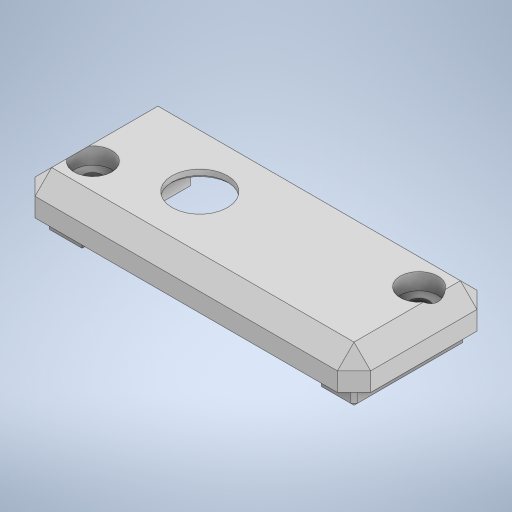
# Autodesk Inventor part: Arm_3_b
Saved by Autodesk Inventor 2023 (Build 270158000, 158)
## iProperties
Created: 2025-02-13
Part Number: Arm_3_b
Material: Generic
Document SubType Name: Modeling
Designer: Swoby
Density: 1 g/cm^3
Appearance: Default
Author: Swoby
Autodesk Inventor part; units mm, degrees
sketch "Sketch1" plane through (0, 0, 0) normal (0, 0, 1) x (1, 0, 0)
  line L0 (0, 0) -> (0, 3.1)
  line L1 (0, 3.1) -> (-5, 3.1)
  line L2 (-5, 3.1) -> (-5, 1.5)
  line L3 (-5, 1.5) -> (-7.4, 1.5)
  line L4 (-7.4, 1.5) -> (-7.4, 0)
  line L5 (-7.4, 0) -> (0, 0)
  line L6 (-7.4, 0) -> (-10.65, 0)
  line L7 (-10.65, 0) -> (-10.65, -7.1)
  line L8 (-10.65, -7.1) -> (-18.15, -7.1)
  line L9 (-18.15, -7.1) -> (-18.15, -10.8)
  line L10 (-18.15, -10.8) -> (-10.65, -10.8)
  line L11 (-10.65, -10.8) -> (-10.65, -31.3)
  line L12 (-10.65, -31.3) -> (-20.15, -31.3)
  line L13 (-20.15, -31.3) -> (-20.15, -36.7)
  line L14 (-20.15, -36.7) -> (-10.65, -36.7)
  line L15 (-10.65, -36.7) -> (-10.65, -40.6)
  line L16 (-10.65, -40.6) -> (30.95, -40.6)
  line L17 (30.95, -40.6) -> (30.95, -10.8)
  line L18 (30.95, -10.8) -> (38.45, -10.8)
  line L19 (38.45, -10.8) -> (38.45, -7.1)
  line L20 (38.45, -7.1) -> (30.95, -7.1)
  line L21 (30.95, 0) -> (0, 0)
  line L22 (30.95, 0) -> (30.95, -7.1)
  line L23 (-20.15, -31.3) -> (-20.15, 3.1)
  line L24 (-20.15, 3.1) -> (-5, 3.1)
  line L25 (-20.15, -36.7) -> (-20.15, -43.1)
  line L26 (-20.15, -43.1) -> (40.45, -43.1)
  line L27 (40.45, -43.1) -> (40.45, 3.1)
  line L28 (40.45, 3.1) -> (0, 3.1)
  line L29 (0, -40.6) -> (-2.5, -40.6)
  line L30 (-2.5, -40.6) -> (-2.5, -43.1)
  line L31 (-2.5, -43.1) -> (0, -43.1)
  line L32 (0, -43.1) -> (0, -40.6)
  dimension "d0" = 3.1
  dimension "d2" = 1.6
  dimension "d3" = 14.8
  dimension "d4" = 10
  dimension "d5" = 10.65
  dimension "d6" = 7.1
  dimension "d7" = 7.5
  dimension "d8" = 7.5
  dimension "d9" = 3.7
  dimension "d10" = 3.9
  dimension "d11" = 5.4
  dimension "d12" = 41.6
  dimension "d13" = 40.6
  dimension "d14" = 2
  dimension "d15" = 2.5
  dimension "d16" = 2.5
  dimension "d17" = 2
  constraints: 66 end point, 19 perpendicular, 15 point on line, 3 collinear, 3 horizontal, 2 parallel, 2 vertical
  measures "d0" distance of L0.start L0.end
  measures "d2" distance of L1.end L2.end
  measures "d3" diameter of L4 L0
  measures "d4" diameter of L2 L0
  measures "d5" distance from line of L0.start L7
  measures "d6" distance of L6.end L7.end
  measures "d7" distance of L7.end L8.end
  measures "d8" distance of L19.end L20.end
  measures "d9" distance of L8.end L9.end
  measures "d10" distance of L14.end L15.end
  measures "d11" distance of L12.end L13.end
  measures "d12" distance of L15.end L16.end
  measures "d13" distance between parallel lines of L16 L21
  measures "d14" distance between parallel lines of L23 L9
  measures "d15" distance between parallel lines of L26 L16
  measures "d16" distance between parallel lines of L32 L30
  measures "d17" distance between parallel lines of L27 L19
extrude "Extrusion1" add sketch "Sketch1" along normal mid plane 21.2 contours L5 L4 L3 L2 L1 L0 | L0 L28 L27 L26 L32 L16 L17 L18 L19 L20 L22 L21 | L6 L7 L8 L9 L10 L11 L12 L23 L24 L2 L3 L4 | L26 L30 L16 L32 | L14 L15 L16 L30 L26 L25
sketch "Sketch2" plane through (0, 0, 10.6) normal (0, 0, 1) x (1, 0, 0)
  line L0 (-20.15, -43.1) -> (40.45, -43.1) projected
  line L1 (40.45, -43.1) -> (40.45, 3.1) projected
  line L2 (40.45, 3.1) -> (-20.15, 3.1) projected
  line L3 (-20.15, 3.1) -> (-20.15, -31.3) projected
  line L4 (-20.15, -31.3) -> (-10.65, -31.3) projected
  line L5 (-10.65, -31.3) -> (-10.65, -10.8) projected
  line L6 (-10.65, -10.8) -> (-18.15, -10.8) projected
  line L7 (-18.15, -10.8) -> (-18.15, -7.1) projected
  line L8 (-18.15, -7.1) -> (-10.65, -7.1) projected
  line L9 (-10.65, -7.1) -> (-10.65, 0) projected
  line L10 (-10.65, 0) -> (30.95, 0) projected
  line L11 (30.95, 0) -> (30.95, -7.1) projected
  line L12 (30.95, -7.1) -> (38.45, -7.1) projected
  line L13 (38.45, -7.1) -> (38.45, -10.8) projected
  line L14 (38.45, -10.8) -> (30.95, -10.8) projected
  line L15 (30.95, -10.8) -> (30.95, -40.6) projected
  line L16 (30.95, -40.6) -> (-10.65, -40.6) projected
  line L17 (-10.65, -40.6) -> (-10.65, -36.7) projected
  line L18 (-10.65, -36.7) -> (-20.15, -36.7) projected
  line L19 (-20.15, -36.7) -> (-20.15, -43.1) projected
  line L20 (-20.15, 3.1) -> (40.45, 3.1)
  line L21 (40.45, 3.1) -> (40.45, -43.1)
  line L22 (40.45, -43.1) -> (-20.15, -43.1)
  line L23 (-20.15, -43.1) -> (-20.15, 3.1)
  point P0 (0, 0)
  constraints: 8 end point, 2 parallel, 1 horizontal, 1 perpendicular
extrude "Extrusion2" add sketch "Sketch2" along normal blind 2
mirror "Mirror1" about plane through (0, 0, 0) normal (0, 0, 1) of "Extrusion2"
revolve "Revolution1" cut sketch "Sketch1" angle 360 about axis through (0, 0, 0) along (0, 1, 0) contours L5 L4 L3 L2 L1 L0 | L26 L30 L16 L32
sketch "Sketch3" plane through (0, 0, 0) normal (0, 0, 1) x (1, 0, 0)
  circle A0 centre (70.45, -20) radius 3.4
  line L0 (40.45, -43.1) -> (40.45, 3.1) projected
  line L1 (70.45, -20) -> (40.45, -20) construction
  line L2 (70.45, -20) -> (83.1779, -7.2721) construction
  line L3 (70.45, -20) -> (83.1779, -32.7279) construction
  arc A1 (84.8107, -8.4271) -> (84.5921, -5.8579) centre (83.1779, -7.2721) ccw
  arc A2 (84.5921, -34.1421) -> (84.8107, -31.5729) centre (83.1779, -32.7279) ccw
  line L4 (-20.15, -43.1) -> (40.45, -43.1) construction
  line L5 (75.0462, -15.4038) -> (77.8746, -18.2322) construction
  line L6 (75.0462, -24.5962) -> (77.8746, -21.7678) construction
  line L7 (84.8107, -31.5729) -> (77.8746, -21.7678)
  line L8 (77.8746, -18.2322) -> (84.8107, -8.4271)
  arc A3 (77.8746, -18.2322) -> (77.8746, -21.7678) centre (80.3736, -20) ccw
  line L9 (83.1779, -7.2721) -> (84.5921, -5.8579) construction
  line L10 (83.1779, -32.7279) -> (84.5921, -34.1421) construction
  circle A4 centre (82.1173, -8.3327) radius 0.5
  arc A5 (58.8771, -5.6393) -> (56.3079, -5.8579) centre (57.7221, -7.2721) ccw
  line L11 (68.6822, -12.5754) -> (58.8771, -5.6393)
  arc A6 (68.6822, -12.5754) -> (72.2178, -12.5754) centre (70.45, -10.0764) ccw
  line L12 (82.0229, -5.6393) -> (72.2178, -12.5754)
  arc A7 (84.5921, -5.8579) -> (82.0229, -5.6393) centre (83.1779, -7.2721) ccw
  circle A8 centre (58.7827, -8.3327) radius 0.5
  arc A9 (56.0893, -31.5729) -> (56.3079, -34.1421) centre (57.7221, -32.7279) ccw
  line L13 (63.0254, -21.7678) -> (56.0893, -31.5729)
  arc A10 (63.0254, -21.7678) -> (63.0254, -18.2322) centre (60.5264, -20) ccw
  line L14 (56.0893, -8.4271) -> (63.0254, -18.2322)
  arc A11 (56.3079, -5.8579) -> (56.0893, -8.4271) centre (57.7221, -7.2721) ccw
  circle A12 centre (58.7827, -31.6673) radius 0.5
  arc A13 (82.0229, -34.3607) -> (84.5921, -34.1421) centre (83.1779, -32.7279) ccw
  line L15 (72.2178, -27.4246) -> (82.0229, -34.3607)
  arc A14 (72.2178, -27.4246) -> (68.6822, -27.4246) centre (70.45, -29.9236) ccw
  line L16 (58.8771, -34.3607) -> (68.6822, -27.4246)
  arc A15 (56.3079, -34.1421) -> (58.8771, -34.3607) centre (57.7221, -32.7279) ccw
  circle A16 centre (82.1173, -31.6673) radius 0.5
  line L17 (40.45, -3.2793) -> (87.1779, -3.2793)
  line L18 (87.1779, -3.2793) -> (87.1779, -36.7279)
  line L19 (87.1779, -36.7279) -> (40.45, -36.7279)
  line L20 (40.45, -36.7279) -> (40.45, -3.2793) construction
  circle A17 centre (70.45, -20) radius 2.25
  point P0 (0, 0)
  point P1 (57.5526, -5.2793)
  point P2 (84.5921, -5.8579)
  point P3 (56.3079, -5.8579)
  dimension "d23" = 6.8
  dimension "d24" = 4
  dimension "d25" = 4
  dimension "d26" = 135
  dimension "d28" = 46.2
  dimension "d29" = 23.1
  dimension "d30" = 18
  dimension "d31" = 18
  dimension "d32" = 4
  dimension "d33" = 4
  dimension "d34" = 6.5
  dimension "d35" = 6.5
  dimension "d36" = 1
  dimension "d37" = 1.5
  dimension "d40" = 360
  dimension "d42" = 2
  dimension "d43" = 4
  dimension "d44" = 4
  dimension "d45" = 4.5
  dimension "d95" = 30
  constraints: 38 end point, 25 point on circle, 18 centre point, 5 perpendicular, 4 point on line, 3 coincident, 3 tangent, 2 collinear, 2 parallel, 1 horizontal, 1 midpoint, 65 other
  measures "d23" diameter of A0
  measures "d24" diameter of A1
  measures "d25" diameter of A2
  measures "d26" angle of L1 L2
  measures "d28" distance of L0.start L0.end
  measures "d29" distance between parallel lines of L4 L1
  measures "d30" distance of L1.start L2.end
  measures "d31" distance of L1.start L3.end
  measures "d32" distance of L5.start L5.end
  measures "d33" distance of L6.start L6.end
  measures "d34" distance between parallel lines of L3 L5
  measures "d35" distance between parallel lines of L2 L6
  measures "d36" diameter of A4
  measures "d37" distance of L2.end A4.centre
  measures "d42" distance from line of point (57.553, -5.279) L17
  measures "d43" distance from line of L18 L9.start
  measures "d44" distance from line of L19 A15.centre
  measures "d45" diameter of A17
  measures "d95" distance from line of L0 L1.start
ref_plane "Work Plane1" through (0, 0, 23.8) normal (0, 0, 1) x (1, 0, 0)
extrude "Extrusion3" add sketch "Sketch3" along normal blind 6 from surface at 23.8 contours A0 | L0 L17 L18 L19 | L8 A3 L7 A2 A13 L15 A14 L16 A15 A9 L13 A10 L14 A11 A5 L11 A6 L12 A7 A1 | A4 | A8 | A12 | A16 | A17
sketch "Sketch4" plane through (40.45, -3.2793, 29.8) normal (0, 1, 0) x (1, 0, 0)
  circle A0 centre (-40.45, 29.8) radius 5 projected
  line L0 (-60.6, 42.4) -> (-60.6, 17.2) projected
  line L1 (0, 17.2) -> (-60.6, 17.2) projected
  line L2 (0, 42.4) -> (0, 17.2) projected
  line L3 (0, 42.4) -> (-60.6, 42.4) projected
  line L4 (0, 0) -> (46.7279, 0) projected
  line L5 (46.7279, 0) -> (46.7279, 6) projected
  line L6 (0, 6) -> (46.7279, 6) projected
  line L7 (0, 6) -> (0, 0) projected
  line L8 (0, 6) -> (0, 17.2)
  line L9 (0, 0) -> (-6, 0)
  line L10 (-6, 0) -> (-6, 17.2)
  dimension "d49" = 6
  constraints: 6 end point, 2 point on line, 1 collinear, 1 horizontal, 1 perpendicular
  measures "d49" distance between parallel lines of L8 L10
extrude "Extrusion4" add sketch "Sketch4" against normal up to surface (33.4486 mm away) contours L1 L8 L7 L9 L10
chamfer "Chamfer2" distance 4 angle 45 2 edges at (34.45, -20.0036, 29.8) (40.45, -20.0036, 23.8)
chamfer "Chamfer3" distance 4 angle 45 2 edges at (87.1779, -3.2793, 26.8) (87.1779, -36.7279, 26.8)
mirror "Mirror3" about plane through (0, 0, 0) normal (0, 0, 1) of "Extrusion3", "Chamfer3", "Chamfer2", "Extrusion4"
chamfer "Chamfer4" distance 20 distance2 6 1 edges at (34.45, -20.0036, 12.6) measured on face at (-1.95, -14.4264, 12.6)
chamfer "Chamfer5" distance 20 distance2 6 1 edges at (34.45, -20.0036, -12.6) measured on face at (-1.95, -14.4264, -12.6)
chamfer "Chamfer6" distance 3 angle 45 14 edges at (10.15, 3.1, 12.6) (40.45, 3.1, 0) (10.15, 3.1, -12.6) (-20.15, 3.1, 0) (-20.15, -20, 12.6) (10.15, -43.1, 12.6) (10.15, -43.1, -12.6) (-20.15, -43.1, 0) (40.45, -43.1, 0) (-20.15, -20, -12.6) (40.45, -39.914, -12.6) (40.45, -0.0896, -12.6) (40.45, -0.0896, 12.6) (40.45, -39.914, 12.6)
chamfer "Chamfer7" distance 2 angle 45 33 edges at (40.45, -3.2793, 14.7) (42.45, -3.2793, 21.8) (34.45, -20.0036, 18.6) (24.45, -3.2793, 15.6) (34.45, -3.2793, 22.2) (36.45, -3.2793, 27.8) (60.814, -3.2793, 29.8) (63.814, -3.2793, 23.8) (85.1779, -5.2793, 23.8) (87.1779, -20.0036, 23.8) (63.814, -36.7279, 23.8) (85.1779, -34.7279, 23.8) (42.45, -36.7279, 21.8) (36.45, -36.7279, 27.8) (34.45, -36.7279, 22.2) (24.45, -36.7279, 15.6) (40.45, -36.7279, 14.7) (40.45, -36.7279, -14.7) (42.45, -36.7279, -21.8) (63.814, -36.7279, -23.8) (24.45, -36.7279, -15.6) (34.45, -36.7279, -22.2) (36.45, -36.7279, -27.8) (85.1779, -34.7279, -23.8) (87.1779, -20.0036, -23.8) (85.1779, -5.2793, -23.8) (63.814, -3.2793, -23.8) (60.814, -3.2793, -29.8) (24.45, -3.2793, -15.6) (40.45, -3.2793, -14.7) (42.45, -3.2793, -21.8) (34.45, -3.2793, -22.2) (36.45, -3.2793, -27.8)
extrude "Extrusion5" cut sketch "Sketch3" along normal blind 6 from surface at 23.8 contours A0 | A4 | A8 | A12 | A16 | A17
extrude "Extrusion6" cut sketch "Sketch3" along normal blind 4 from surface at 23.8 contours L8 A3 L7 A2 A13 L15 A14 L16 A15 A9 L13 A10 L14 A11 A5 L11 A6 L12 A7 A1
extrude "Extrusion7" add sketch "Sketch3" along normal blind 2.5 from surface at -23.8 contours A17
ref_plane "Work Plane2" through (48.664, -3.2793, -12.6) normal (0, 1, 0) x (-1, 0, 0)
sketch "Sketch5" plane through (48.664, -3.2793, -12.6) normal (0, 1, 0) x (-1, 0, 0)
  line L0 (59.314, 2) -> (17.714, 2) projected
  line L1 (17.714, 2) -> (17.714, 23.2) projected
  line L2 (17.714, 23.2) -> (59.314, 23.2) projected
  line L3 (59.314, 2) -> (59.314, 23.2) projected
  line L4 (68.814, 3) -> (68.814, 22.2) projected
  line L5 (65.814, 0) -> (68.814, 3) projected
  line L6 (65.814, 0) -> (11.214, 0) projected
  line L7 (68.814, 22.2) -> (65.814, 25.2) projected
  line L8 (11.214, 25.2) -> (65.814, 25.2) projected
  line L9 (12.214, -4.5119) -> (27.2538, 0) projected
  line L10 (12.214, -12.3716) -> (12.214, -4.5119) projected
  line L11 (9.3855, -15.2) -> (12.214, -12.3716) projected
  line L12 (-34.514, -15.2) -> (9.3855, -15.2) projected
  line L13 (-34.514, -13.2) -> (-34.514, -15.2) projected
  line L14 (5.0424, -13.2) -> (-34.514, -13.2) projected
  line L15 (10.214, -8.0284) -> (5.0424, -13.2) projected
  line L16 (10.214, 1) -> (10.214, -8.0284) projected
  line L17 (11.214, 0) -> (10.214, 1) projected
  line L18 (27.2538, 0) -> (11.214, 0) projected
  line L19 (12.214, 29.7119) -> (12.214, 37.5716) projected
  line L20 (27.2538, 25.2) -> (12.214, 29.7119) projected
  line L21 (11.214, 25.2) -> (27.2538, 25.2) projected
  line L22 (10.214, 24.2) -> (11.214, 25.2) projected
  line L23 (10.214, 33.2284) -> (10.214, 24.2) projected
  line L24 (5.0424, 38.4) -> (10.214, 33.2284) projected
  line L25 (-34.514, 38.4) -> (5.0424, 38.4) projected
  line L26 (-34.514, 40.4) -> (-34.514, 38.4) projected
  line L27 (9.3855, 40.4) -> (-34.514, 40.4) projected
  line L28 (12.214, 37.5716) -> (9.3855, 40.4) projected
  line L29 (8.214, 3) -> (8.214, 22.2) projected
  line L30 (10.214, 1) -> (8.214, 3) projected
  line L31 (8.214, 22.2) -> (10.214, 24.2) projected
  circle A0 centre (13.964, 7.7) radius 1.75
  circle A1 centre (13.964, 7.7) radius 2.15
  circle A2 centre (13.964, 7.7) radius 3.4
  circle A3 centre (63.064, 17.5) radius 1.75
  circle A4 centre (63.064, 17.5) radius 2.15
  circle A5 centre (63.064, 17.5) radius 3.4
  line L32 (66.814, 2) -> (66.814, 23.2) projected
  line L33 (59.314, 23.2) -> (66.814, 23.2) projected
  line L34 (59.314, 2) -> (59.314, 23.2) projected
  line L35 (66.814, 2) -> (59.314, 2) projected
  line L36 (17.714, 2) -> (17.714, 23.2) projected
  line L37 (10.214, 23.2) -> (17.714, 23.2) projected
  line L38 (10.214, 2) -> (10.214, 23.2) projected
  line L39 (17.714, 2) -> (10.214, 2) projected
  point P0 (48.664, 12.6)
  point P1 (66.814, 12.6)
  point P2 (8.214, 12.6)
  dimension "d79" = 3.5
  dimension "d80" = 4.3
  dimension "d81" = 6.8
  dimension "d82" = 3.5
  dimension "d83" = 4.3
  dimension "d84" = 6.8
  dimension "d101" = 4.9
  dimension "d105" = 4.9
  dimension "d123" = 7.5
  dimension "d124" = 3.75
  dimension "d125" = 7.5
  dimension "d126" = 3.75
  constraints: 6 centre point, 3 coincident, 2 midpoint, 1 concentric
  measures "d79" diameter of A0
  measures "d80" diameter of A1
  measures "d81" diameter of A2
  measures "d82" diameter of A3
  measures "d83" diameter of A4
  measures "d84" diameter of A5
  measures "d101" vertical distance of A3.centre point (66.814, 12.6)
  measures "d105" vertical distance of point (8.214, 12.6) A0.centre
  measures "d123" distance between parallel lines of L3 L32
  measures "d124" distance from line of L32 A3.centre
  measures "d125" distance of L36.start L38.start
  measures "d126" distance from line of L38 A0.centre
extrude "Extrusion9" cut sketch "Sketch5" against normal blind 3 from surface at 6.3793 contours A0 | A1 | A2 | A3 | A4 | A5
extrude "Extrusion10" cut sketch "Sketch5" along normal through all contours A0 | A3
extrude "Extrusion11" cut sketch "Sketch5" against normal blind 16 contours A0 | A1 | A3 | A4
extrude "Extrusion12" cut sketch "Sketch5" against normal up to surface (3.8207 mm away) contours L3 L33 L32 L35 | L39 L38 L37 L1 | A0 | A1 | A2 | A3 | A4 | A5
ref_plane "Work Plane3" through (70.1779, -32.7279, -27.8) normal (1, 0, 0) x (0, 0, -1)
sketch "Sketch6" plane through (70.1779, -32.7279, -27.8) normal (1, 0, 0) x (0, 0, -1)
  line L0 (2, 24.6202) -> (2, 27.4486) projected
  line L1 (2, 0.8284) -> (2, 24.6202) projected
  line L2 (2, -2) -> (2, 0.8284) projected
  line L3 (2, 27.4486) -> (2, -2) projected
  line L4 (2, 12.7243) -> (4, 12.7243) construction
  line L5 (4, 15.2243) -> (4, 10.2243)
  line L6 (4, 10.2243) -> (2, 8.5461)
  line L7 (4, 10.2243) -> (7.0319, 10.2243) construction
  line L8 (4, 15.2243) -> (2, 16.9025)
  line L9 (4, 15.2243) -> (7.6595, 15.2243) construction
  line L10 (2, 6.588) -> (5.5, 9.5249)
  line L11 (5.5, 9.5249) -> (5.5, 15.9238)
  line L12 (5.5, 15.9238) -> (2, 18.8606)
  point P0 (-27.8, 32.7279)
  point P1 (2, 8.5461)
  point P2 (2, 16.9025)
  dimension "d107" = 2
  dimension "d108" = 5
  dimension "d109" = 140
  dimension "d110" = 140
  dimension "d111" = 1.5
  dimension "d112" = 1.5
  dimension "d113" = 1.5
  constraints: 18 end point, 4 point on line, 3 horizontal, 2 midpoint, 2 parallel, 2 vertical
  measures "d107" distance of L4.end L4.start
  measures "d108" distance of L5.start L5.end
  measures "d109" angle of L6 L7
  measures "d110" angle of L9 L8
  measures "d111" distance between parallel lines of L10 L6
  measures "d112" distance between parallel lines of L11 L5
  measures "d113" distance between parallel lines of L12 L8
extrude "Extrusion13" add sketch "Sketch6" along normal mid plane 3 contours L1 L6 L5 L8 L12 L11 L10
split "Split1" plane through (48.664, -3.2793, -12.6) removes the side toward (0, -1, 0)
sketch "Sketch7" plane through (48.664, -3.2793, -12.6) normal (0, -1, 0) x (1, 0, 0)
  line L0 (-10.214, 2) -> (-10.214, 23.2) projected
  line L1 (-10.214, 23.2) -> (-17.714, 23.2) projected
  line L2 (-17.714, 2) -> (-17.714, 23.2) projected
  line L3 (-17.714, 2) -> (-10.214, 2) projected
  circle A0 centre (-13.964, 7.7) radius 1.75 projected
  circle A1 centre (-63.064, 17.5) radius 1.75 projected
  line L4 (-66.814, 2) -> (-66.814, 23.2) projected
  line L5 (-59.314, 23.2) -> (-66.814, 23.2) projected
  line L6 (-59.314, 23.2) -> (-59.314, 2) projected
  line L7 (-66.814, 2) -> (-59.314, 2) projected
  line L8 (-17.214, 2) -> (-17.214, 22.7)
  line L9 (-17.214, 22.7) -> (-10.714, 22.7)
  line L10 (-10.714, 22.7) -> (-10.714, 2.5)
  line L11 (-10.714, 2.5) -> (-17.714, 2.5)
  line L12 (-59.814, 2) -> (-59.814, 22.7)
  line L13 (-59.814, 22.7) -> (-66.314, 22.7)
  line L14 (-66.314, 22.7) -> (-66.314, 2.5)
  line L15 (-66.314, 2.5) -> (-59.314, 2.5)
  point P0 (-48.664, 12.6)
  point P1 (-59.814, 2.5)
  point P2 (-17.214, 2.5)
  dimension "d116" = 0.5
  dimension "d117" = 0.5
  constraints: 16 end point, 6 other
  measures "d116" distance between parallel lines of L0 L10
  measures "d117" distance between parallel lines of L6 L12
extrude "Extrusion14" add sketch "Sketch7" along normal blind 3.6 contours L8 L9 L10 L11 | L15 L14 L13 L12
chamfer "Chamfer8" distance 0.6 angle 45 17 edges at (-17.65, -5.0793, 10.1) (-17.65, -6.8793, 0) (-14.4, -6.8793, 10.1) (-11.15, -6.8793, 0) (-17.65, -5.0793, -10.1) (-14.4, -6.8793, -10.1) (-11.15, -5.0793, -10.1) (31.45, -5.0793, -10.1) (34.7, -6.8793, -10.1) (31.45, -6.8793, 0) (37.95, -6.8793, 0) (37.95, -5.0793, -10.1) (31.45, -5.0793, 10.1) (34.7, -6.8793, 10.1) (37.95, -5.0793, 10.1) (7.4, 0, 0) (5, 1.5, 0)
equation "\"d8\" = d7"
equation "\"d29\" = 0.5 * d28"
equation "\"d31\" = d30"
equation "\"d105\" = d101"
body "Solid1"
